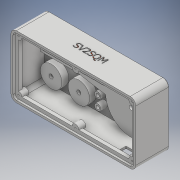
# Autodesk Inventor part: box
Saved by Autodesk Inventor 2017.3 (Build 213257000, 257)
## iProperties
Created: 2021-12-05
Part Number: box
Material: Generic
Document SubType Name: Modeling
Designer: TEOS
Density: 1 g/cm^3
Appearance: Default
Author: TEOS
Autodesk Inventor part; units mm, degrees
ref_plane "YZ Plane" through (0, 0, 0) normal (1, 0, 0) x (0, 1, 0)
ref_plane "XZ Plane" through (0, 0, 0) normal (0, 1, 0) x (-1, 0, 0)
sketch "Sketch1" plane through (0, 0, 0) normal (0, 1, 0) x (-1, 0, 0)
  line L0 (82, -45) -> (-82, -45)
  line L1 (-90, -37) -> (-90, 37)
  line L2 (-82, 45) -> (82, 45)
  line L3 (90, 37) -> (90, -37)
  arc A0 (82, -45) -> (90, -37) centre (82, -37) ccw
  arc A1 (90, 37) -> (82, 45) centre (82, 37) ccw
  arc A2 (-90, -37) -> (-82, -45) centre (-82, -37) ccw
  arc A3 (-82, 45) -> (-90, 37) centre (-82, 37) ccw
  line L4 (-82, -42) -> (82, -42)
  arc A4 (82, -42) -> (87, -37) centre (82, -37) ccw
  line L5 (87, -37) -> (87, 37)
  arc A5 (87, 37) -> (82, 42) centre (82, 37) ccw
  line L6 (82, 42) -> (-82, 42)
  arc A6 (-82, 42) -> (-87, 37) centre (-82, 37) ccw
  line L7 (-87, 37) -> (-87, -37)
  arc A7 (-87, -37) -> (-82, -42) centre (-82, -37) ccw
  point P0 (0, 0)
  point P1 (90, -45)
  point P2 (-90, -45)
  point P3 (90, 45)
  dimension "d0" = 180
  dimension "d1" = 90
  dimension "d2" = 8
  dimension "d3" = 3
  dimension "d24" = 90
  dimension "d25" = 45
  constraints: 16 end point, 16 point on circle, 8 centre point, 8 tangent, 6 point on line, 4 parallel, 3 equal radius, 2 perpendicular, 1 horizontal, 7 other
  measures "d0" distance of point (90, -45) point (-90, -45)
  measures "d1" distance of point (90, 45) point (90, -45)
  measures "d2" radius of A0
  measures "d3" distance between parallel lines of L0 L4
  measures "d24" distance from line of L1 point (0, 0)
  measures "d25" distance from line of point (0, 0) L0
extrude "Extrusion1" add sketch "Sketch1" along normal blind 45
sketch "Sketch2" plane through (0, 45, 0) normal (0, 1, 0) x (1, 0, 0)
  line L0 (82, 45) -> (-82, 45)
  arc A0 (-82, 45) -> (-90, 37) centre (-82, 37) ccw
  line L1 (-90, 37) -> (-90, -37)
  arc A1 (-90, -37) -> (-82, -45) centre (-82, -37) ccw
  line L2 (-82, -45) -> (82, -45)
  arc A2 (82, -45) -> (90, -37) centre (82, -37) ccw
  line L3 (90, -37) -> (90, 37)
  arc A3 (90, 37) -> (82, 45) centre (82, 37) ccw
  circle A4 centre (48.5, 3.5) radius 34
  circle A5 centre (-67, 22) radius 12.5
  circle A6 centre (-27, 22) radius 12.5
  line L4 (-90, 22) -> (90, 22) construction
  line L5 (20.5, -25.065714) -> (20.5, -34.5)
  line L6 (20.5, -34.5) -> (-79.5, -34.5)
  line L7 (-79.5, -34.5) -> (-79.5, -4.5)
  arc A7 (9.308164, -4.5) -> (20.5, -25.065714) centre (48.5, 3.5) ccw
  line L8 (-79.5, -4.5) -> (9.308164, -4.5)
  line L9 (-29.5, -4.5) -> (-29.5, -34.5)
  line L10 (-33.5, -4.5) -> (-33.5, -34.5)
  line L11 (-25.5, -4.5) -> (-25.5, -34.5)
  point P0 (0, 0)
  dimension "d6" = 68
  dimension "d7" = 41.5
  dimension "d8" = 41.5
  dimension "d9" = 25
  dimension "d10" = 25
  dimension "d11" = 23
  dimension "d12" = 23
  dimension "d13" = 40
  dimension "d14" = 100
  dimension "d15" = 30
  dimension "d16" = 10.5
  dimension "d17" = 10.5
  dimension "d18" = 80
  dimension "d19" = 50
  dimension "d20" = 8
  dimension "d21" = 4
  constraints: 16 end point, 9 point on line, 4 centre point, 4 perpendicular, 2 parallel, 2 point on circle, 1 coincident, 1 horizontal, 1 midpoint
  measures "d6" diameter of A4
  measures "d7" distance from line of L3 A4.centre
  measures "d8" distance from line of L0 A4.centre
  measures "d9" diameter of A6
  measures "d10" diameter of A5
  measures "d11" distance between parallel lines of L0 L4
  measures "d12" distance of A5.centre L4.start
  measures "d13" distance of A6.centre A5.centre
  measures "d14" distance of L5.end L6.end
  measures "d15" distance of L6.end L7.end
  measures "d16" distance between parallel lines of L7 L1
  measures "d17" distance between parallel lines of L2 L6
  measures "d18" diameter of A7
  measures "d19" distance between parallel lines of L7 L9
  measures "d20" distance between parallel lines of L11 L10
  measures "d21" distance between parallel lines of L10 L9
extrude "Extrusion2" add sketch "Sketch2" along normal blind 3 contours A3 L3 A2 L2 A1 L1 A0 L0 | L6 L9 L8 L11 | L6 L10 L8 L9
sketch "Sketch3" plane through (0, 45, 0) normal (0, -1, 0) x (1, 0, 0)
  circle A0 centre (-67, -22) radius 12.5
  circle A1 centre (-27, -22) radius 12.5
  line L0 (-25.5, 34.5) -> (20.5, 34.5)
  line L1 (20.5, 34.5) -> (20.5, 25.065714)
  arc A2 (20.5, 25.065714) -> (9.308164, 4.5) centre (48.5, -3.5) ccw
  line L2 (9.308164, 4.5) -> (-25.5, 4.5)
  line L3 (-25.5, 4.5) -> (-25.5, 34.5)
  line L4 (-33.5, 4.5) -> (-79.5, 4.5)
  line L5 (-79.5, 4.5) -> (-79.5, 34.5)
  line L6 (-79.5, 34.5) -> (-33.5, 34.5)
  line L7 (-33.5, 34.5) -> (-33.5, 4.5)
  circle A3 centre (48.5, -3.5) radius 34
  arc A4 (82, -42) -> (87, -37) centre (82, -37) ccw
  line L8 (87, -37) -> (87, 37)
  arc A5 (87, 37) -> (82, 42) centre (82, 37) ccw
  line L9 (82, 42) -> (-82, 42)
  arc A6 (-82, 42) -> (-87, 37) centre (-82, 37) ccw
  line L10 (-87, 37) -> (-87, -37)
  arc A7 (-87, -37) -> (-82, -42) centre (-82, -37) ccw
  line L11 (-82, -42) -> (82, -42)
  circle A8 centre (48.5, -3.5) radius 37
  arc A9 (23.5, 23.776363) -> (11.554094, -5.5) centre (48.5, -3.5) ccw
  line L12 (23.5, 23.776363) -> (23.5, 37.5)
  line L13 (23.5, 37.5) -> (-28.5, 37.5)
  line L14 (-28.5, 1.5) -> (11.554094, -5.5)
  line L15 (-82.5, 1.5) -> (-30.5, 1.5)
  line L16 (-30.5, 37.5) -> (-82.5, 37.5)
  line L17 (-82.5, 37.5) -> (-82.5, 1.5)
  circle A10 centre (-27, -22) radius 15.5
  circle A11 centre (-67, -22) radius 15.5
  line L18 (-28.5, 1.5) -> (-30.5, 1.5)
  line L19 (-28.5, 37.5) -> (-30.5, 37.5)
  point P0 (0, 0)
  dimension "d26" = 3
  dimension "d27" = 3
  dimension "d28" = 3
  dimension "d29" = 3
  dimension "d30" = 3
  constraints: 16 end point, 4 centre point, 2 point on circle, 3 other
  measures "d26" radial gap between concentric circles of A3 A8
  measures "d27" radial gap between concentric circles of A2 A9
  measures "d28" distance between parallel lines of L4 L15
  measures "d29" radial gap between concentric circles of A1 A10
  measures "d30" radial gap between concentric circles of A0 A11
extrude "Extrusion3" add sketch "Sketch3" along normal blind 7 contours A8 | A8 L14 L18 L15 L17 L16 L19 L13 L12 | A10 | A11
sketch "Sketch4" plane through (0, 38, 0) normal (0, -1, 0) x (1, 0, 0)
  circle A0 centre (48.5, -3.5) radius 34
  line L0 (-79.5, 4.5) -> (-79.5, 34.5)
  line L1 (-79.5, 34.5) -> (-33.5, 34.5)
  line L2 (-33.5, 34.5) -> (-33.5, 4.5)
  line L3 (-33.5, 4.5) -> (-79.5, 4.5)
  line L4 (20.5, 34.5) -> (20.5, 25.065714)
  arc A1 (20.5, 25.065714) -> (9.308164, 4.5) centre (48.5, -3.5) ccw
  line L5 (9.308164, 4.5) -> (-25.5, 4.5)
  line L6 (-25.5, 4.5) -> (-25.5, 34.5)
  line L7 (-25.5, 34.5) -> (20.5, 34.5)
  line L8 (23.5, 23.776363) -> (23.5, 37.5)
  line L9 (23.5, 37.5) -> (-82.5, 37.5)
  line L10 (-82.5, 37.5) -> (-82.5, 1.5)
  line L11 (-28.5, 1.5) -> (11.554094, -5.5)
  arc A2 (11.554094, -5.5) -> (23.5, 23.776363) centre (48.5, -3.5) ccw
  circle A3 centre (-27, -22) radius 12.5
  circle A4 centre (-27, -22) radius 15.5
  circle A5 centre (-67, -22) radius 12.5
  circle A6 centre (-67, -22) radius 15.5
  circle A7 centre (48.5, -3.5) radius 37
  line L12 (-82.5, 1.5) -> (-28.5, 1.5)
  point P0 (0, 0)
  constraints: 1 coincident, 3 other
extrude "Extrusion4" add sketch "Sketch4" along normal blind 3 contours A0 | A7 L11 L12 L10 L9 L8 | A2 A7 | A3 | A4 | A5 | A6
sketch "Sketch5" plane through (0, 35, 0) normal (0, -1, 0) x (1, 0, 0)
  circle A0 centre (-27, -22) radius 15.5
  circle A1 centre (-67, -22) radius 15.5
  line L0 (-79.5, 34.5) -> (-33.5, 34.5)
  line L1 (-33.5, 34.5) -> (-33.5, 4.5)
  line L2 (-33.5, 4.5) -> (-79.5, 4.5)
  line L3 (-79.5, 4.5) -> (-79.5, 34.5)
  arc A2 (20.5, 25.065714) -> (9.308164, 4.5) centre (48.5, -3.5) ccw
  line L4 (9.308164, 4.5) -> (-25.5, 4.5)
  line L5 (-25.5, 4.5) -> (-25.5, 34.5)
  line L6 (-25.5, 34.5) -> (20.5, 34.5)
  line L7 (20.5, 34.5) -> (20.5, 25.065714)
  line L8 (23.5, 23.776363) -> (23.5, 37.5)
  line L9 (23.5, 37.5) -> (-82.5, 37.5)
  line L10 (-82.5, 37.5) -> (-82.5, 1.5)
  line L11 (-28.5, 1.5) -> (11.554094, -5.5)
  arc A3 (11.554094, -5.5) -> (23.5, 23.776363) centre (48.5, -3.5) ccw
  line L12 (-82.5, 1.5) -> (-28.5, 1.5)
  point P0 (0, 0)
hole "Hole1" at (48.5, 35, -3.5) at (-27, 35, -22) at (-67, 35, -22) direction (0, 1, 0) diameter 6 end through all
chamfer "Chamfer1" distance 1 angle 45 8 edges at (87.6569, 48, 42.6569) (90, 48, 0) (87.6569, 48, -42.6569) (0, 48, -45) (-87.6569, 48, -42.6569) (-90, 48, 0) (-87.6569, 48, 42.6569) (0, 48, 45)
ref_plane "Work Plane1" through (0, 3, 0) normal (0, -1, 0) x (1, 0, 0)
sketch "Sketch7" plane through (0, 3, 0) normal (0, -1, 0) x (1, 0, 0)
  line L0 (82, -42) -> (-82, -42)
  arc A0 (-82, 42) -> (-87, 37) centre (-82, 37) ccw
  line L1 (-82, -32) -> (-82, 32)
  line L2 (82, 32) -> (82, -32)
  line L3 (82, 42) -> (-82, 42)
  arc A1 (77, 37) -> (82, 32) centre (82, 37) ccw
  arc A2 (82, -32) -> (77, -37) centre (82, -37) ccw
  arc A3 (-82, 32) -> (-77, 37) centre (-82, 37) ccw
  arc A4 (-82, 42) -> (-82.5, 41.974937) centre (-82, 37) ccw
  arc A5 (-86.974937, 37.5) -> (-87, 37) centre (-82, 37) ccw
  arc A6 (-77, -37) -> (-82, -32) centre (-82, -37) ccw
  arc A7 (-83.180286, -41.858696) -> (-82, -42) centre (-82, -37) ccw
  arc A8 (5, -37) -> (-5, -37) centre (0, -37) ccw
  arc A9 (-5, 37) -> (5, 37) centre (0, 37) ccw
  line L4 (77, -37) -> (5, -37)
  line L5 (-5, -37) -> (-77, -37)
  line L6 (-77, 37) -> (-5, 37)
  line L7 (5, 37) -> (77, 37)
  line L8 (87, 37) -> (87, -37)
  arc A10 (82, -42) -> (87, -37) centre (82, -37) ccw
  arc A11 (87, 37) -> (82, 42) centre (82, 37) ccw
  line L9 (-82, 42) -> (82, 42)
  arc A12 (-82, 42) -> (-87, 37) centre (-82, 37) ccw
  line L10 (-87, -37) -> (-87, 37)
  arc A13 (-87, -37) -> (-82, -42) centre (-82, -37) ccw
  circle A14 centre (82, -37) radius 5
  circle A15 centre (-82, -37) radius 5
  point P0 (0, 0)
  dimension "d65" = 5
  dimension "d66" = 5
  dimension "d67" = 5
  dimension "d68" = 5
  constraints: 19 point on circle, 15 end point, 9 centre point, 5 coincident, 5 parallel, 2 horizontal, 2 perpendicular, 2 vertical alignment, 6 other
  measures "d65" distance between parallel lines of L0 L5
  measures "d66" distance between parallel lines of L0 L4
  measures "d67" radius of A8
  measures "d68" distance from line of L0 A8.centre
extrude "Extrusion5" add sketch "Sketch7" against normal blind 10 contours A14 A2 A10 | L0 A15 L5 A8 L4 A14 | A7 A13 A15 A6 | A14 L2 A1 L7 A9 L6 A3 L1 A15 L10 A0 L3 A11 L8
sketch "Sketch8" plane through (0, 3, 0) normal (0, -1, 0) x (1, 0, 0)
  arc A0 (-77, -37) -> (-82, -32) centre (-82, -37) ccw projected
  line L0 (-82, -32) -> (-82, 32) projected
  arc A1 (-82, 32) -> (-77, 37) centre (-82, 37) ccw projected
  line L1 (-77, 37) -> (-5, 37) projected
  arc A2 (-5, 37) -> (5, 37) centre (0, 37) ccw projected
  line L2 (5, 37) -> (77, 37) projected
  arc A3 (77, 37) -> (82, 32) centre (82, 37) ccw projected
  line L3 (82, 32) -> (82, -32) projected
  arc A4 (82, -32) -> (77, -37) centre (82, -37) ccw projected
  line L4 (77, -37) -> (5, -37) projected
  arc A5 (5, -37) -> (-5, -37) centre (0, -37) ccw projected
  line L5 (-5, -37) -> (-77, -37) projected
  line L6 (82, -42) -> (-82, -42) projected
  arc A6 (82, -42) -> (87, -37) centre (82, -37) ccw projected
  line L7 (87, 37) -> (87, -37) projected
  arc A7 (87, 37) -> (82, 42) centre (82, 37) ccw projected
  line L8 (-82, 42) -> (82, 42) projected
  arc A8 (-82, 42) -> (-87, 37) centre (-82, 37) ccw projected
  line L9 (-87, -37) -> (-87, 37) projected
  arc A9 (-87, -37) -> (-82, -42) centre (-82, -37) ccw projected
  arc A10 (5, -37) -> (-5, -37) centre (0, -37) ccw projected
  point P0 (0, 0)
  constraints: 6 coincident
hole "Hole2" at (82, 3, 37) at (0, 3, 37) at (0, 3, -37) at (82, 3, -37) at (-82, 3, -37) at (-82, 3, 37) direction (0, 1, 0) diameter 2 depth 15 tip angle 118
chamfer "Chamfer2" distance 5 angle 45 6 edges at (-41, 13, 37) (41, 13, 37) (82, 13, 0) (41, 13, -37) (-41, 13, -37) (-82, 13, 0)
sketch "Sketch10" plane through (82, 0, -45) normal (0, 0, -1) x (-1, 0, 0)
  line L0 (18.017065, 20) -> (24.017065, 20)
  line L1 (24.017065, 20) -> (26.017065, 18)
  line L2 (26.017065, 18) -> (26.017065, 11)
  line L3 (26.017065, 11) -> (16.017065, 11)
  line L4 (16.017065, 11) -> (16.017065, 18)
  line L5 (16.017065, 18) -> (18.017065, 20)
  line L6 (15.017065, 10) -> (27.017065, 10)
  line L7 (27.017065, 10) -> (27.017065, 21)
  line L8 (15.017065, 21) -> (27.017065, 21)
  line L9 (15.017065, 10) -> (15.017065, 21)
  line L10 (27.017065, 9) -> (15.017065, 9)
  line L11 (14.017065, 10) -> (14.017065, 21)
  line L12 (15.017065, 22) -> (27.017065, 22)
  line L13 (28.017065, 21) -> (28.017065, 10)
  arc A0 (27.017065, 9) -> (28.017065, 10) centre (27.017065, 10) ccw
  arc A1 (28.017065, 21) -> (27.017065, 22) centre (27.017065, 21) ccw
  arc A2 (15.017065, 22) -> (14.017065, 21) centre (15.017065, 21) ccw
  arc A3 (14.017065, 10) -> (15.017065, 9) centre (15.017065, 10) ccw
  point P0 (82, 0)
  dimension "d69" = 1
  dimension "d70" = 1
  constraints: 8 end point, 8 point on circle, 8 tangent, 4 centre point, 3 equal radius, 3 other
  measures "d69" distance between parallel lines of L6 L10
  measures "d70" radius of A0
extrude "Extrusion6" cut sketch "Sketch10" against normal blind 10 contours L0 L1 L2 L3 L4 L5 | L9 L8 L7 L6 | L10 A3 L11 A2 L12 A1 L13 A0
sketch "Sketch11" plane through (-82, 0, 45) normal (0, 0, 1) x (1, 0, 0)
  line L0 (58.91807, 30.223223) -> (103.85932, 30.223223) construction
  line L1 (103.85932, 30.223223) -> (103.85932, 18.984365) construction
  line L2 (103.85932, 18.984365) -> (58.91807, 18.984365) construction
  line L3 (58.91807, 18.984365) -> (58.91807, 30.223223) construction
  line L4 (164, 48) -> (0, 48)
  line L5 (169, 3) -> (164, 3)
  line L6 (0, 48) -> (164, 3)
  line L7 (164, 3) -> (164, 48)
  line L8 (0, 47) -> (164, 47)
  line L9 (164, 48) -> (0, 3)
  spline S0 degree 2 poles (62.243638, 21.132866) (61.293475, 21.132866) (59.960412, 21.529948) (59.371879, 21.813579) knots 0 0 0 1 2 2 2
  line L10 (59.371879, 21.813579) -> (59.371879, 23.274276)
  line L11 (59.371879, 23.274276) -> (59.456968, 23.274276)
  spline S1 degree 2 poles (59.456968, 23.274276) (60.03132, 22.735378) (61.484926, 22.139754) (62.158548, 22.139754) knots 0 0 0 1 2 2 2
  spline S2 degree 2 poles (62.158548, 22.139754) (63.122892, 22.139754) (64.108508, 22.94101) (64.108508, 23.600451) knots 0 0 0 1 2 2 2
  spline S3 degree 2 poles (64.108508, 23.600451) (64.108508, 24.125167) (63.590882, 24.777517) (63.030712, 24.940605) knots 0 0 0 1 2 2 2
  spline S4 degree 2 poles (63.030712, 24.940605) (62.626539, 25.054057) (61.952916, 25.210054) (61.449472, 25.337687) knots 0 0 0 1 2 2 2
  spline S5 degree 2 poles (61.449472, 25.337687) (60.995663, 25.45823) (60.279497, 25.819859) (60.002957, 26.11058) knots 0 0 0 1 2 2 2
  spline S6 degree 2 poles (60.002957, 26.11058) (59.733508, 26.401302) (59.435696, 27.181285) (59.435696, 27.69182) knots 0 0 0 1 2 2 2
  spline S7 degree 2 poles (59.435696, 27.69182) (59.435696, 28.755434) (61.094934, 30.194859) (62.378362, 30.194859) knots 0 0 0 1 2 2 2
  spline S8 degree 2 poles (62.378362, 30.194859) (63.115801, 30.194859) (64.420501, 29.904138) (64.980672, 29.627598) knots 0 0 0 1 2 2 2
  line L12 (64.980672, 29.627598) -> (64.980672, 28.237809)
  line L13 (64.980672, 28.237809) -> (64.895582, 28.237809)
  spline S9 degree 2 poles (64.895582, 28.237809) (64.477228, 28.62071) (63.172527, 29.187971) (62.45636, 29.187971) knots 0 0 0 1 2 2 2
  spline S10 degree 2 poles (62.45636, 29.187971) (61.648014, 29.187971) (60.648216, 28.429259) (60.648216, 27.812363) knots 0 0 0 1 2 2 2
  spline S11 degree 2 poles (60.648216, 27.812363) (60.648216, 27.259284) (61.236749, 26.599843) (61.789829, 26.450937) knots 0 0 0 1 2 2 2
  spline S12 degree 2 poles (61.789829, 26.450937) (62.158548, 26.351666) (63.229253, 26.096399) (63.583792, 25.990037) knots 0 0 0 1 2 2 2
  spline S13 degree 2 poles (63.583792, 25.990037) (64.484318, 25.713498) (65.321028, 24.600248) (65.321028, 23.78481) knots 0 0 0 1 2 2 2
  spline S14 degree 2 poles (65.321028, 23.78481) (65.321028, 23.267185) (64.902673, 22.274478) (64.526863, 21.927031) knots 0 0 0 1 2 2 2
  spline S15 degree 2 poles (64.526863, 21.927031) (64.108508, 21.54413) (63.044894, 21.132866) (62.243638, 21.132866) knots 0 0 0 1 2 2 2
  line L14 (72.851417, 30.038862) -> (69.837843, 21.288862)
  line L15 (69.837843, 21.288862) -> (68.582779, 21.288862)
  line L16 (68.582779, 21.288862) -> (65.569205, 30.038862)
  line L17 (65.569205, 30.038862) -> (66.817179, 30.038862)
  line L18 (66.817179, 30.038862) -> (69.242219, 22.770832)
  line L19 (69.242219, 22.770832) -> (71.66726, 30.038862)
  line L20 (71.66726, 30.038862) -> (72.851417, 30.038862)
  line L21 (78.83602, 21.288862) -> (73.43995, 21.288862)
  line L22 (73.43995, 21.288862) -> (73.43995, 22.529746)
  spline S16 degree 2 poles (73.43995, 22.529746) (74.021393, 23.075734) (75.056644, 24.089713) (75.552997, 24.635702) knots 0 0 0 1 2 2 2
  spline S17 degree 2 poles (75.552997, 24.635702) (76.552795, 25.73477) (77.283143, 27.053652) (77.283143, 27.755637) knots 0 0 0 1 2 2 2
  spline S18 degree 2 poles (77.283143, 27.755637) (77.283143, 28.124357) (77.056239, 28.677436) (76.850607, 28.854705) knots 0 0 0 1 2 2 2
  spline S19 degree 2 poles (76.850607, 28.854705) (76.644975, 29.031974) (76.106077, 29.209243) (75.779902, 29.209243) knots 0 0 0 1 2 2 2
  spline S20 degree 2 poles (75.779902, 29.209243) (75.467908, 29.209243) (74.82974, 29.053246) (74.539018, 28.932704) knots 0 0 0 1 2 2 2
  spline S21 degree 2 poles (74.539018, 28.932704) (74.290842, 28.833433) (73.829942, 28.549802) (73.688127, 28.450532) knots 0 0 0 1 2 2 2
  line L23 (73.688127, 28.450532) -> (73.62431, 28.450532)
  line L24 (73.62431, 28.450532) -> (73.62431, 29.698506)
  spline S22 degree 2 poles (73.62431, 29.698506) (73.985939, 29.875775) (75.283548, 30.223222) (75.864991, 30.223222) knots 0 0 0 1 2 2 2
  spline S23 degree 2 poles (75.864991, 30.223222) (77.091693, 30.223222) (78.474391, 28.925613) (78.474391, 27.819454) knots 0 0 0 1 2 2 2
  spline S24 degree 2 poles (78.474391, 27.819454) (78.474391, 27.301828) (78.233305, 26.436755) (78.020582, 26.068036) knots 0 0 0 1 2 2 2
  spline S25 degree 2 poles (78.020582, 26.068036) (77.80786, 25.685135) (77.190963, 24.933514) (76.850607, 24.571885) knots 0 0 0 1 2 2 2
  spline S26 degree 2 poles (76.850607, 24.571885) (76.297527, 23.96917) (74.943192, 22.678652) (74.539018, 22.302841) knots 0 0 0 1 2 2 2
  line L25 (74.539018, 22.302841) -> (78.83602, 22.302841)
  line L26 (78.83602, 22.302841) -> (78.83602, 21.288862)
  spline S27 degree 2 poles (82.693394, 21.132866) (81.743232, 21.132866) (80.410169, 21.529948) (79.821636, 21.813579) knots 0 0 0 1 2 2 2
  line L27 (79.821636, 21.813579) -> (79.821636, 23.274276)
  line L28 (79.821636, 23.274276) -> (79.906725, 23.274276)
  spline S28 degree 2 poles (79.906725, 23.274276) (80.481077, 22.735378) (81.934683, 22.139754) (82.608305, 22.139754) knots 0 0 0 1 2 2 2
  spline S29 degree 2 poles (82.608305, 22.139754) (83.572649, 22.139754) (84.558265, 22.94101) (84.558265, 23.600451) knots 0 0 0 1 2 2 2
  spline S30 degree 2 poles (84.558265, 23.600451) (84.558265, 24.125167) (84.040639, 24.777517) (83.480469, 24.940605) knots 0 0 0 1 2 2 2
  spline S31 degree 2 poles (83.480469, 24.940605) (83.076296, 25.054057) (82.402673, 25.210054) (81.899229, 25.337687) knots 0 0 0 1 2 2 2
  spline S32 degree 2 poles (81.899229, 25.337687) (81.44542, 25.45823) (80.729253, 25.819859) (80.452714, 26.11058) knots 0 0 0 1 2 2 2
  spline S33 degree 2 poles (80.452714, 26.11058) (80.183265, 26.401302) (79.885453, 27.181285) (79.885453, 27.69182) knots 0 0 0 1 2 2 2
  spline S34 degree 2 poles (79.885453, 27.69182) (79.885453, 28.755434) (81.544691, 30.194859) (82.828119, 30.194859) knots 0 0 0 1 2 2 2
  spline S35 degree 2 poles (82.828119, 30.194859) (83.565558, 30.194859) (84.870258, 29.904138) (85.430428, 29.627598) knots 0 0 0 1 2 2 2
  line L29 (85.430428, 29.627598) -> (85.430428, 28.237809)
  line L30 (85.430428, 28.237809) -> (85.345339, 28.237809)
  spline S36 degree 2 poles (85.345339, 28.237809) (84.926984, 28.62071) (83.622284, 29.187971) (82.906117, 29.187971) knots 0 0 0 1 2 2 2
  spline S37 degree 2 poles (82.906117, 29.187971) (82.09777, 29.187971) (81.097973, 28.429259) (81.097973, 27.812363) knots 0 0 0 1 2 2 2
  spline S38 degree 2 poles (81.097973, 27.812363) (81.097973, 27.259284) (81.686506, 26.599843) (82.239586, 26.450937) knots 0 0 0 1 2 2 2
  spline S39 degree 2 poles (82.239586, 26.450937) (82.608305, 26.351666) (83.67901, 26.096399) (84.033548, 25.990037) knots 0 0 0 1 2 2 2
  spline S40 degree 2 poles (84.033548, 25.990037) (84.934075, 25.713498) (85.770785, 24.600248) (85.770785, 23.78481) knots 0 0 0 1 2 2 2
  spline S41 degree 2 poles (85.770785, 23.78481) (85.770785, 23.267185) (85.35243, 22.274478) (84.97662, 21.927031) knots 0 0 0 1 2 2 2
  spline S42 degree 2 poles (84.97662, 21.927031) (84.558265, 21.54413) (83.494651, 21.132866) (82.693394, 21.132866) knots 0 0 0 1 2 2 2
  spline S43 degree 2 poles (94.222973, 19.147452) (93.903889, 19.069454) (93.208994, 18.984365) (92.861547, 18.984365) knots 0 0 0 1 2 2 2
  spline S44 degree 2 poles (92.861547, 18.984365) (91.875931, 18.984365) (90.649229, 20.083433) (90.592503, 21.104503) knots 0 0 0 1 2 2 2
  spline S45 degree 2 poles (90.592503, 21.104503) (90.514505, 21.104503) (90.37978, 21.104503) (90.323054, 21.104503) knots 0 0 0 1 2 2 2
  spline S46 degree 2 poles (90.323054, 21.104503) (89.436709, 21.104503) (88.011466, 21.707217) (87.500931, 22.295751) knots 0 0 0 1 2 2 2
  spline S47 degree 2 poles (87.500931, 22.295751) (86.997487, 22.877193) (86.458589, 24.578976) (86.458589, 25.656772) knots 0 0 0 1 2 2 2
  spline S48 degree 2 poles (86.458589, 25.656772) (86.458589, 26.76293) (87.004578, 28.43635) (87.508022, 29.031974) knots 0 0 0 1 2 2 2
  spline S49 degree 2 poles (87.508022, 29.031974) (88.018557, 29.620507) (89.4438, 30.223222) (90.323054, 30.223222) knots 0 0 0 1 2 2 2
  spline S50 degree 2 poles (90.323054, 30.223222) (91.21649, 30.223222) (92.648824, 29.599235) (93.145177, 29.031974) knots 0 0 0 1 2 2 2
  spline S51 degree 2 poles (93.145177, 29.031974) (93.641531, 28.457622) (94.19461, 26.748749) (94.19461, 25.656772) knots 0 0 0 1 2 2 2
  spline S52 degree 2 poles (94.19461, 25.656772) (94.19461, 23.954989) (92.868638, 21.742671) (91.712843, 21.352679) knots 0 0 0 1 2 2 2
  spline S53 degree 2 poles (91.712843, 21.352679) (91.741206, 21.026504) (91.911385, 20.501788) (92.046109, 20.352882) knots 0 0 0 1 2 2 2
  spline S54 degree 2 poles (92.046109, 20.352882) (92.209197, 20.168522) (92.655915, 19.998344) (93.052997, 19.998344) knots 0 0 0 1 2 2 2
  spline S55 degree 2 poles (93.052997, 19.998344) (93.286993, 19.998344) (93.925161, 20.14725) (94.066976, 20.203976) knots 0 0 0 1 2 2 2
  line L31 (94.066976, 20.203976) -> (94.222973, 20.203976)
  line L32 (94.222973, 20.203976) -> (94.222973, 19.147452)
  spline S56 degree 2 poles (92.98209, 25.656772) (92.98209, 26.528935) (92.606279, 27.869089) (92.265923, 28.308716) knots 0 0 0 1 2 2 2
  spline S57 degree 2 poles (92.265923, 28.308716) (91.918475, 28.762525) (90.93995, 29.216334) (90.330145, 29.216334) knots 0 0 0 1 2 2 2
  spline S58 degree 2 poles (90.330145, 29.216334) (89.699067, 29.216334) (88.748905, 28.776707) (88.387276, 28.308716) knots 0 0 0 1 2 2 2
  spline S59 degree 2 poles (88.387276, 28.308716) (88.039829, 27.861999) (87.671109, 26.507663) (87.671109, 25.656772) knots 0 0 0 1 2 2 2
  spline S60 degree 2 poles (87.671109, 25.656772) (87.671109, 23.933716) (89.117625, 22.097209) (90.330145, 22.097209) knots 0 0 0 1 2 2 2
  spline S61 degree 2 poles (90.330145, 22.097209) (91.542665, 22.097209) (92.98209, 23.933716) (92.98209, 25.656772) knots 0 0 0 1 2 2 2
  line L33 (102.972973, 21.288862) -> (101.810088, 21.288862)
  line L34 (101.810088, 21.288862) -> (101.810088, 28.826342)
  line L35 (101.810088, 28.826342) -> (99.526863, 23.699721)
  line L36 (99.526863, 23.699721) -> (98.817787, 23.699721)
  line L37 (98.817787, 23.699721) -> (96.555834, 28.826342)
  line L38 (96.555834, 28.826342) -> (96.555834, 21.288862)
  line L39 (96.555834, 21.288862) -> (95.470947, 21.288862)
  line L40 (95.470947, 21.288862) -> (95.470947, 30.038862)
  line L41 (95.470947, 30.038862) -> (97.059278, 30.038862)
  line L42 (97.059278, 30.038862) -> (99.243232, 25.167509)
  line L43 (99.243232, 25.167509) -> (101.356279, 30.038862)
  line L44 (101.356279, 30.038862) -> (102.972973, 30.038862)
  line L45 (102.972973, 30.038862) -> (102.972973, 21.288862)
  point P0 (82, 0)
  constraints: 6 end point, 1 perpendicular, 2 other
emboss "Emboss1" sketch "Sketch11" operation cut depth 1.5 direction (0, 0, -1) contours L42 L43 L44 L45 L33 L34 L35 L36 L37 L38 L6 L40 L9 | L9 L40 L41 L42 | L16 L17 L18 L6 | L6 L18 L19 L14 L9 L16 | L38 L39 L40 L6 | L9 L14 L15 L16 | S51 S52 L6 S61 S56 S57 L9 | L9 S57 S58 S59 S48 S49 S50 S51 | L19 L20 L14 L6 | S52 S53 S54 S55 L31 L32 S43 S44 S45 S46 S47 L6 S60 S61 | S16 S17 L6 S24 S25 S26 L9 | L9 S26 L25 L26 L21 L22 S16 | S59 S60 L6 S47 S48 L9 | S17 S18 S19 S20 S21 L23 L24 S22 S23 S24 L6 | S32 L6 L9 | L9 L6 S40 S41 S42 S27 L27 L28 S28 S29 S30 S31 S32 | S39 S40 L6 L9 | L9 L6 S32 S33 S34 S35 L29 L30 S36 S37 S38 S39 | S0 L10 L11 S1 S2 S3 S4 S5 S6 S7 S8 L12 L13 S9 S10 S11 S12 S13 S14 S15
sketch "Sketch12" plane through (0, 45, 0) normal (0, -1, 0) x (1, 0, 0)
  circle A0 centre (-67, -22) radius 3 construction
  circle A1 centre (0, -12) radius 4.5
  circle A2 centre (0, -27) radius 4.5
  circle A3 centre (0, -12) radius 2.45
  circle A4 centre (0, -27) radius 2.45
  arc A5 (5, -37) -> (-5, -37) centre (0, -37) ccw
  line L0 (0, -37) -> (0, -6.169334)
  point P0 (0, 0)
  dimension "d75" = 9
  dimension "d76" = 9
  dimension "d77" = 4.9
  dimension "d78" = 4.9
  dimension "d79" = 15
  dimension "d81" = 10
  constraints: 4 centre point, 2 coincident, 2 end point, 2 point on line, 1 vertical
  measures "d75" diameter of A1
  measures "d76" diameter of A2
  measures "d77" diameter of A3
  measures "d78" diameter of A4
  measures "d79" distance of A2.centre A1.centre
  measures "d81" distance of L0.start A2.centre
extrude "Extrusion7" add sketch "Sketch12" along normal blind 10 contours A1 L0 A3 | L0 A3 A1 | A2 L0 A4 | L0 A4 A2
body "Solid1"
